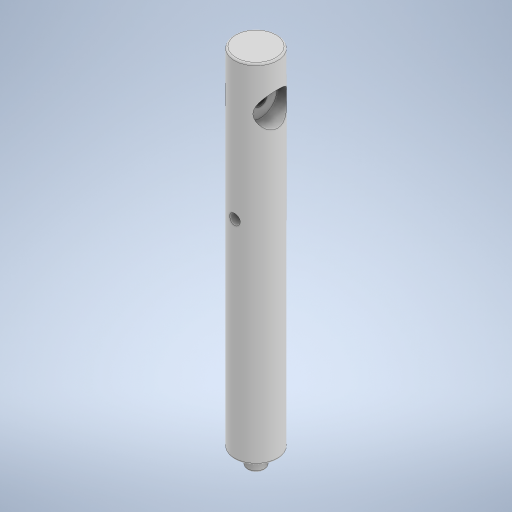
# Autodesk Inventor part: CorpoRedondo_6_193_5_249_motor_furo99_2
Saved by Autodesk Inventor 2023.2 (Build 272271030, 271C)
## iProperties
Created: 2023-04-15
Part Number: CorpoRedondo_6_193_5_249_motor_furo99_2
Material: Generic
Document SubType Name: Modeling
Designer: victo
Density: 1 g/cm^3
Appearance: Default
Author: victo
## iProperties of the stored document CorpoRedondo_6_19_5_245_motor_furo_3DPrint.ipt
Created: 2023-05-16
Part Number: CorpoRedondo_6_19_5_245_motor_furo_3DPrint
Material: Generic
Document SubType Name: Modeling
Designer: VICTOR
Density: 1 g/cm^3
Appearance: Default
Author: VICTOR
Autodesk Inventor part; units mm, degrees
note: some values were not read from the file. Chosen so that the rebuilt part matches the saved one: second side of "Extrusion3".
ref_plane "YZ Plane" through (0, 0, 0) normal (1, 0, 0) x (0, 1, 0)
ref_plane "XZ Plane" through (0, 0, 0) normal (0, 1, 0) x (-1, 0, 0)
ref_plane "XY Plane" through (0, 0, 0) normal (0, 0, 1) x (1, 0, 0)
sketch "Sketch1" plane through (0, 0, 0) normal (0, 1, 0) x (-1, 0, 0)
  circle A0 centre (0, 0) radius 12.425
  dimension "d0" = 24.85
  constraints: 1 centre point, 1 coincident
  measures "d0" diameter of A0
extrude "Extrusion1" add sketch "Sketch1" along normal blind 200
sketch "Sketch6" plane through (0, 0, 0) normal (1, 0, 0) x (0, 1, 0)
  line L0 (200, 9.25) -> (200, -9.25) projected
  line L1 (200, 0) -> (175, 0)
  circle A0 centre (175, 0) radius 9.65
  line L2 (0, 12.425) -> (200, 12.425) projected
  line L3 (0, -12.425) -> (200, -12.425) projected
  line L4 (0, 12.425) -> (200, 12.425) projected
  point P0 (0, 0)
  dimension "d7" = 25
  dimension "d8" = 19.3
  constraints: 2 end point, 1 centre point, 1 coincident, 1 horizontal, 1 midpoint
  measures "d7" distance of L1.start L1.end
  measures "d8" diameter of A0
extrude "Extrusion3" add sketch "Sketch6" along normal blind 12.45
sketch "Sketch8" plane through (12.45, 175, 0) normal (1, 0, 0) x (0, 0, -1)
  circle A0 centre (0, 0) radius 9.65 projected
  point P0 (0, -175)
extrude "Extrusion4" cut sketch "Sketch8" against normal blind 10
sketch "Sketch9" plane through (2.45, 175, 0) normal (1, 0, 0) x (0, 0, -1)
  circle A0 centre (0, 0) radius 3.9
  point P0 (0, -175)
  dimension "d16" = 7.8
  constraints: 1 centre point
  measures "d16" diameter of A0
extrude "Extrusion5" cut sketch "Sketch9" along normal mid plane 15
sketch "Sketch10" plane through (0, 0, 0) normal (0, -1, 0) x (1, 0, 0)
  circle A0 centre (0, 0) radius 4.95
  dimension "d19" = 9.9
  constraints: 1 centre point, 1 coincident
  measures "d19" diameter of A0
extrude "Extrusion6" add sketch "Sketch10" along normal blind 9
sketch "Sketch11" plane through (0, -9, 0) normal (0, -1, 0) x (1, 0, 0)
  circle A0 centre (0, 0) radius 2.6
  dimension "d22" = 5.2
  constraints: 1 centre point, 1 coincident
  measures "d22" diameter of A0
extrude "Extrusion7" cut sketch "Sketch11" against normal blind 10
sketch "Sketch12" plane through (0, 0, 0) normal (0, 0, 1) x (1, 0, 0)
  line L0 (12.425, 200) -> (-12.425, 200) projected
  line L1 (12.425, 0) -> (-12.425, 0) projected
  line L2 (0, 200) -> (0, 120)
  circle A0 centre (0, 120) radius 3.05
  point P0 (0, 0)
  point P1 (7.8268, 175)
  dimension "d25" = 80
  dimension "d28" = 6.1
  constraints: 2 end point, 1 centre point, 1 coincident, 1 midpoint, 1 vertical
  measures "d25" distance of L2.start L2.end
  measures "d28" diameter of A0
extrude "Extrusion8" add sketch "Sketch12" along normal blind 24.5
sketch "Sketch13" plane through (0, 120, 24.5) normal (0, 0, 1) x (1, 0, 0)
  circle A0 centre (0, 0) radius 3.05 projected
  point P0 (0, -120)
extrude "Extrusion9" cut sketch "Sketch13" against normal blind 50
fillet "Fillet4" radius 1 3 edges at (12.425, 200, 0) (12.425, 0, 0) (-4.95, -9, 0)
extrude "Extrusion10" add sketch "Sketch6" against normal blind 12.45
sketch "Sketch15" plane through (-12.45, 175, 0) normal (-1, 0, 0) x (0, 0, 1)
  circle A0 centre (0, 0) radius 3.9 projected
  circle A1 centre (0, 0) radius 9.65 projected
  point P0 (0, -175)
extrude "Extrusion11" cut sketch "Sketch15" against normal blind 150 contours A0
sketch "Sketch16" plane through (-12.45, 175, 0) normal (-1, 0, 0) x (0, 0, 1)
  circle A0 centre (0, 0) radius 3.9 projected
  circle A1 centre (0, 0) radius 9.65 projected
  point P0 (0, -175)
extrude "Extrusion12" cut sketch "Sketch16" against normal blind 10
body "Solid1"
